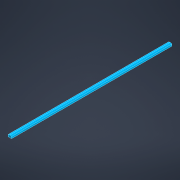
# Autodesk Inventor part: CentreBackCushion
Saved by Autodesk Inventor 2021 (Build 250183000, 183)
## iProperties
Created: 2021-01-30
Part Number: CentreBackCushion
Material: Generic
Document SubType Name: Modeling
Designer: argon
Density: 1 g/cm^3
Appearance: Sky Blue Medium
Author: argon
Autodesk Inventor part; units mm, degrees
ref_plane "YZ Plane" through (0, 0, 0) normal (1, 0, 0) x (0, 1, 0)
ref_plane "XZ Plane" through (0, 0, 0) normal (0, 1, 0) x (-1, 0, 0)
ref_plane "XY Plane" through (0, 0, 0) normal (0, 0, 1) x (1, 0, 0)
sketch "Sketch1" plane through (0, 0, 0) normal (0, 0, 1) x (1, 0, 0)
  line L0 (0, 12.8132) -> (5.7633, 12.8132) construction
  line L1 (5.7633, 12.8132) -> (10, 10) construction
  spline S0 degree 2 poles (0, 12.8132) (5.7633, 12.8132) (10, 10) knots 1 1 1 2 2 2
  line L2 (0, 0) -> (10, 0)
  line L3 (10, 0) -> (10, 10)
  line L4 (0, 13.9209) -> (0, -2.5018) construction
  line L5 (0, 12.8132) -> (-5.7633, 12.8132) construction
  line L6 (-5.7633, 12.8132) -> (-10, 10) construction
  spline S1 degree 2 poles (0, 12.8132) (-5.7633, 12.8132) (-10, 10) knots 1 1 1 2 2 2
  line L7 (0, 0) -> (-10, 0)
  line L8 (-10, 0) -> (-10, 10)
  dimension "d0" = 10
  dimension "d1" = 10
  constraints: 10 end point, 3 symmetric about line, 1 horizontal, 1 perpendicular, 1 vertical, 6 other
  measures "d0" distance of L2.start L2.end
  measures "d1" distance of L2.end L1.end
extrude "Extrusion1" add sketch "Sketch1" along normal blind 900
body "Solid1"
